Autodesk Fusion 360 part; units mm, degrees
(part 3 of 23)
  arc A1021 (27.2288, 53.8875) -> (27.2288, 53.8367) centre (27.2288, 53.8621) ccw
  arc A1022 (31.8008, 2.5146) -> (31.8008, 2.4638) centre (31.8008, 2.4892) ccw
  arc A1023 (65.6214, 47.9446) -> (65.5634, 47.994) centre (65.5924, 47.9693) ccw
  arc A1024 (33.504, 1.5804) -> (33.4532, 1.5804) centre (33.4786, 1.5804) ccw
  arc A1025 (34.1907, 2.4638) -> (34.1907, 2.5146) centre (34.1907, 2.4892) ccw
  arc A1026 (34.4504, 2.4638) -> (34.4504, 2.5146) centre (34.4504, 2.4892) ccw
  arc A1027 (32.4499, 2.4638) -> (32.4499, 2.5146) centre (32.4499, 2.4892) ccw
  arc A1028 (33.219, 1.3462) -> (33.219, 1.2954) centre (33.219, 1.3208) ccw
  arc A1029 (33.4532, 1.5804) -> (33.504, 1.5804) centre (33.4786, 1.5804) ccw
  arc A1030 (65.766, 48.2854) -> (65.6898, 48.2854) centre (65.7279, 48.2854) ccw
  arc A1031 (65.7279, 47.0281) -> (65.7279, 47.1043) centre (65.7279, 47.0662) ccw
  arc A1032 (32.8873, 2.2296) -> (32.8366, 2.2296) centre (32.862, 2.2296) ccw
  line L321 (64.8248, 47.0662) -> (65.7279, 47.0662)
  arc A1033 (33.3366, 1.7853) -> (33.3609, 1.8299) centre (33.3488, 1.8076) ccw
  line L322 (34.4504, 1.3208) -> (34.1907, 1.3208)
  arc A1034 (64.8248, 47.1043) -> (64.8248, 47.0281) centre (64.8248, 47.0662) ccw
  arc A1035 (33.9565, 2.2296) -> (33.9057, 2.2296) centre (33.9311, 2.2296) ccw
  arc A1036 (32.9789, 1.9805) -> (33.0047, 2.0242) centre (32.9918, 2.0023) ccw
  arc A1037 (33.1216, 2.4892) -> (32.862, 2.2296) centre (33.1216, 2.2296) ccw
  arc A1038 (33.4786, 1.5804) -> (33.3488, 1.8076) centre (33.2149, 1.5804) ccw
  arc A1039 (34.1907, 1.2954) -> (34.1907, 1.3462) centre (34.1907, 1.3208) ccw
  arc A1040 (32.1, 1.3208) -> (32.1508, 1.3208) centre (32.1254, 1.3208) ccw
  arc A1041 (33.219, 1.2954) -> (33.219, 1.3462) centre (33.219, 1.3208) ccw
  arc A1042 (33.1216, 2.5146) -> (33.1216, 2.4638) centre (33.1216, 2.4892) ccw
  arc A1043 (33.9057, 1.5804) -> (33.9565, 1.5804) centre (33.9311, 1.5804) ccw
  arc A1044 (33.9057, 2.2296) -> (33.9565, 2.2296) centre (33.9311, 2.2296) ccw
  arc A1045 (34.1907, 2.4892) -> (33.9311, 2.2296) centre (34.1907, 2.2296) ccw
  line L323 (34.1907, 2.4892) -> (34.4504, 2.4892)
  arc A1046 (34.871, 2.2494) -> (34.9028, 2.2097) centre (34.8869, 2.2295) ccw
  line L324 (34.8869, 2.2296) -> (35.2114, 2.4892)
  arc A1047 (35.2368, 2.4892) -> (35.186, 2.4892) centre (35.2114, 2.4892) ccw
  arc A1048 (32.8475, 1.501) -> (32.8115, 1.4652) centre (32.8295, 1.4831) ccw
  arc A1049 (32.8366, 2.2296) -> (32.8873, 2.2296) centre (32.862, 2.2296) ccw
  arc A1050 (34.8869, 1.3462) -> (34.8869, 1.2954) centre (34.8869, 1.3208) ccw
  line L325 (32.1254, 1.3208) -> (32.1254, 2.4892)
  line L326 (36.0299, 2.2296) -> (36.3544, 2.4892)
  line L327 (65.5924, 47.9693) -> (64.8248, 47.0662)
  line L328 (34.8869, 1.3208) -> (35.536, 1.3208)
  arc A1051 (36.3703, 2.4694) -> (36.3386, 2.509) centre (36.3544, 2.4892) ccw
  arc A1052 (36.014, 2.2494) -> (36.0458, 2.2097) centre (36.0299, 2.2295) ccw
  line L329 (31.8008, 2.4892) -> (32.4499, 2.4892)
  arc A1053 (33.9311, 1.5804) -> (34.1907, 1.3208) centre (34.1907, 1.5804) ccw
  arc A1054 (33.1216, 2.4638) -> (33.1216, 2.5146) centre (33.1216, 2.4892) ccw
  arc A1055 (33.3985, 2.3715) -> (33.4289, 2.4122) centre (33.4137, 2.3918) ccw
  line L330 (33.3488, 1.8076) -> (32.9918, 2.0024)
  arc A1056 (35.2273, 2.4694) -> (35.1956, 2.509) centre (35.2114, 2.4892) ccw
  line L331 (36.3544, 2.4892) -> (36.3544, 1.3208)
  arc A1057 (34.4504, 1.2954) -> (34.4504, 1.3462) centre (34.4504, 1.3208) ccw
  arc A1058 (33.219, 1.3208) -> (33.4786, 1.5804) centre (33.219, 1.5804) ccw
  arc A1059 (64.7957, 47.0909) -> (64.8538, 47.0415) centre (64.8247, 47.0662) ccw
  arc A1060 (32.1508, 2.4892) -> (32.1, 2.4892) centre (32.1254, 2.4892) ccw
  line L332 (33.9311, 1.5804) -> (33.9311, 2.2296)
  arc A1061 (53.8714, 1.9445) -> (53.8714, 1.9953) centre (53.8714, 1.9699) ccw
  arc A1062 (34.1907, 1.3462) -> (34.1907, 1.2954) centre (34.1907, 1.3208) ccw
  line L333 (54.9481, 1.3208) -> (54.6885, 1.3208)
  arc A1063 (33.0039, 2.0247) -> (32.9796, 1.9801) centre (32.9917, 2.0024) ccw
  arc A1064 (33.4137, 2.3918) -> (33.1216, 2.4892) centre (33.1216, 2.0024) ccw
  arc A1065 (34.1907, 2.5146) -> (34.1907, 2.4638) centre (34.1907, 2.4892) ccw
  arc A1066 (35.186, 1.3208) -> (35.2368, 1.3208) centre (35.2114, 1.3208) ccw
  arc A1067 (35.536, 1.2954) -> (35.536, 1.3462) centre (35.536, 1.3208) ccw
  arc A1068 (32.862, 2.2296) -> (32.9918, 2.0024) centre (33.1257, 2.2296) ccw
  arc A1069 (33.3617, 1.8295) -> (33.3359, 1.7857) centre (33.3488, 1.8076) ccw
  arc A1070 (32.8295, 1.4831) -> (33.219, 1.3208) centre (33.219, 1.8694) ccw
  arc A1071 (33.9565, 1.5804) -> (33.9057, 1.5804) centre (33.9311, 1.5804) ccw
  line L334 (35.2114, 2.4892) -> (35.2114, 1.3208)
  line L335 (59.134, 11.2155) -> (57.706, 11.7348)
  line L336 (34.2251, 29.7505) -> (34.8742, 29.1987)
  arc A1072 (33.9576, 29.1745) -> (33.9733, 29.2229) centre (33.9655, 29.1987) ccw
  line L337 (55.633, 1.3208) -> (55.633, 2.4892)
  arc A1073 (26.6305, 29.6644) -> (26.5797, 29.6644) centre (26.6051, 29.6644) ccw
  arc A1074 (50.9947, 29.8986) -> (50.9947, 29.9494) centre (50.9947, 29.924) ccw
  arc A1075 (55.6584, 2.4892) -> (55.6076, 2.4892) centre (55.633, 2.4892) ccw
  arc A1076 (58.9788, 10.1219) -> (59.0296, 10.1219) centre (59.0042, 10.1219) ccw
  arc A1077 (59.1253, 11.1916) -> (59.1427, 11.2394) centre (59.134, 11.2155) ccw
  arc A1078 (57.8499, 14.0955) -> (57.8217, 14.0533) centre (57.8358, 14.0744) ccw
  arc A1079 (59.0156, 12.8511) -> (58.9928, 12.8966) centre (59.0042, 12.8739) ccw
  arc A1080 (58.9901, 13.2743) -> (59.0183, 13.3166) centre (59.0042, 13.2954) ccw
  arc A1081 (36.679, 1.2954) -> (36.679, 1.3462) centre (36.679, 1.3208) ccw
  arc A1082 (57.8217, 13.3166) -> (57.8499, 13.2743) centre (57.8358, 13.2954) ccw
  arc A1083 (60.3758, 8.9662) -> (60.3758, 8.9154) centre (60.3758, 8.9408) ccw
  arc A1084 (60.7004, 9.5899) -> (60.3758, 9.2654) centre (60.7004, 9.2653) ccw
  arc A1085 (58.5103, 12.5493) -> (58.4595, 12.5493) centre (58.4849, 12.5493) ccw
  arc A1086 (57.8104, 12.2248) -> (57.8612, 12.2248) centre (57.8358, 12.2248) ccw
  line L338 (54.6885, 2.4892) -> (54.9481, 2.4892)
  arc A1087 (57.8104, 12.5493) -> (57.8612, 12.5493) centre (57.8358, 12.5493) ccw
  line L339 (58.4849, 12.5493) -> (58.4849, 12.2248)
  line L340 (59.0042, 12.2248) -> (57.8358, 12.2248)
  line L341 (61.5442, 8.9408) -> (60.3758, 8.9408)
  arc A1088 (60.7004, 9.5645) -> (60.7004, 9.6153) centre (60.7004, 9.5899) ccw
  arc A1089 (54.6885, 1.2954) -> (54.6885, 1.3462) centre (54.6885, 1.3208) ccw
  arc A1090 (53.4819, 1.9953) -> (53.4819, 1.9445) centre (53.4819, 1.9699) ccw
  arc A1091 (60.3504, 9.2654) -> (60.4012, 9.2654) centre (60.3758, 9.2654) ccw
  line L342 (60.7004, 9.5899) -> (61.2196, 9.5899)
  arc A1092 (60.3504, 8.9408) -> (60.4012, 8.9408) centre (60.3758, 8.9408) ccw
  arc A1093 (50.9947, 29.924) -> (50.7351, 29.6644) centre (50.9947, 29.6644) ccw
  arc A1094 (59.0042, 12.1994) -> (59.0042, 12.2502) centre (59.0042, 12.2248) ccw
  arc A1095 (54.4034, 2.2296) -> (54.4542, 2.2296) centre (54.4288, 2.2296) ccw
  arc A1096 (34.2067, 29.7329) -> (34.2435, 29.768) centre (34.2251, 29.7505) ccw
  arc A1097 (58.4849, 12.5493) -> (57.8358, 12.5493) centre (58.1604, 12.5493) ccw
  arc A1098 (26.5797, 29.6644) -> (26.6305, 29.6644) centre (26.6051, 29.6644) ccw
  arc A1099 (61.5188, 9.2654) -> (61.5696, 9.2654) centre (61.5442, 9.2654) ccw
  arc A1100 (36.3798, 2.4892) -> (36.329, 2.4892) centre (36.3544, 2.4892) ccw
  arc A1101 (60.7004, 9.6153) -> (60.7004, 9.5645) centre (60.7004, 9.5899) ccw
  arc A1102 (60.5492, 10.2421) -> (60.5269, 10.1964) centre (60.5381, 10.2192) ccw
  arc A1103 (60.4012, 9.2654) -> (60.3504, 9.2654) centre (60.3758, 9.2654) ccw
  arc A1104 (61.2196, 9.5645) -> (61.2196, 9.6153) centre (61.2196, 9.5899) ccw
  line L343 (57.8358, 12.2248) -> (57.8358, 12.5493)
  arc A1105 (57.8612, 12.5493) -> (57.8104, 12.5493) centre (57.8358, 12.5493) ccw
  line L344 (59.0042, 12.8739) -> (58.4849, 12.6142)
  arc A1106 (33.6978, 28.4044) -> (33.7138, 28.3562) centre (33.7058, 28.3803) ccw
  line L345 (61.5442, 9.2654) -> (61.5442, 8.9408)
  arc A1107 (33.9979, 29.8224) -> (33.9979, 29.8732) centre (33.9979, 29.8478) ccw
  line L346 (60.3758, 8.9408) -> (60.3758, 9.2654)
  arc A1108 (33.7312, 29.5557) -> (33.6804, 29.5557) centre (33.7058, 29.5557) ccw
  arc A1109 (61.5442, 8.9154) -> (61.5442, 8.9662) centre (61.5442, 8.9408) ccw
  arc A1110 (34.2251, 29.7505) -> (33.9979, 29.8478) centre (33.998, 29.5341) ccw
  arc A1111 (33.7058, 29.5557) -> (33.9654, 29.1987) centre (34.081, 29.5557) ccw
  line L347 (57.8358, 13.2955) -> (59.0042, 14.0744)
  arc A1112 (61.5188, 8.9408) -> (61.5696, 8.9408) centre (61.5442, 8.9408) ccw
  arc A1113 (57.7147, 11.7587) -> (57.6973, 11.7109) centre (57.706, 11.7348) ccw
  arc A1114 (58.4595, 12.5493) -> (58.5103, 12.5493) centre (58.4849, 12.5493) ccw
  arc A1115 (58.4736, 12.6369) -> (58.4963, 12.5915) centre (58.4849, 12.6142) ccw
  arc A1116 (61.5442, 9.2654) -> (61.2196, 9.5899) centre (61.2196, 9.2653) ccw
  arc A1117 (59.0296, 10.771) -> (58.9788, 10.771) centre (59.0042, 10.771) ccw
  arc A1118 (58.4595, 12.2248) -> (58.5103, 12.2248) centre (58.4849, 12.2248) ccw
  line L348 (59.0042, 13.2955) -> (57.8358, 14.0744)
  arc A1119 (57.8358, 12.2502) -> (57.8358, 12.1994) centre (57.8358, 12.2248) ccw
  arc A1120 (59.0183, 14.0533) -> (58.9901, 14.0955) centre (59.0042, 14.0744) ccw
  arc A1121 (61.2196, 9.6153) -> (61.2196, 9.5645) centre (61.2196, 9.5899) ccw
  arc A1122 (60.3504, 10.4464) -> (60.4012, 10.4465) centre (60.3758, 10.4465) ccw
  arc A1123 (61.3737, 10.2433) -> (61.3902, 10.1952) centre (61.382, 10.2192) ccw
  arc A1124 (60.3504, 12.1031) -> (60.4012, 12.1031) centre (60.3758, 12.1031) ccw
  arc A1125 (61.5301, 13.0838) -> (61.5583, 13.1261) centre (61.5442, 13.105) ccw
  arc A1126 (43.4975, 9.6224) -> (43.4467, 9.6224) centre (43.4721, 9.6224) ccw
  arc A1127 (61.5696, 10.4464) -> (61.5188, 10.4465) centre (61.5442, 10.4465) ccw
  arc A1128 (60.6513, 10.7259) -> (60.6196, 10.6863) centre (60.6354, 10.7061) ccw
  arc A1129 (60.2547, 11.7587) -> (60.2373, 11.7109) centre (60.246, 11.7348) ccw
  arc A1130 (60.4012, 12.7522) -> (60.3504, 12.7522) centre (60.3758, 12.7522) ccw
  line L349 (60.3758, 13.105) -> (61.5442, 13.8839)
  arc A1131 (42.6212, 10.4733) -> (42.5704, 10.4733) centre (42.5958, 10.4733) ccw
  line L350 (61.5442, 13.105) -> (60.3758, 13.8839)
  arc A1132 (61.3931, 10.1964) -> (61.3708, 10.2421) centre (61.382, 10.2192) ccw
  arc A1133 (60.96, 10.7456) -> (60.96, 10.7964) centre (60.96, 10.771) ccw
  arc A1134 (60.5381, 10.2193) -> (60.96, 10.1219) centre (60.9601, 11.0846) ccw
  arc A1135 (60.96, 10.0965) -> (60.96, 10.1473) centre (60.96, 10.1219) ccw
  arc A1136 (61.6653, 11.1916) -> (61.6827, 11.2394) centre (61.674, 11.2155) ccw
  arc A1137 (61.3708, 10.6508) -> (61.3931, 10.6965) centre (61.382, 10.6737) ccw
  line L351 (61.5442, 12.4276) -> (60.3758, 12.4276)
  arc A1138 (61.5583, 13.8628) -> (61.5301, 13.905) centre (61.5442, 13.8839) ccw
  arc A1139 (60.5381, 10.6736) -> (60.3758, 10.4465) centre (60.6159, 10.4465) ccw
  arc A1140 (60.3617, 13.1261) -> (60.3899, 13.0838) centre (60.3758, 13.1049) ccw
  line L352 (43.4721, 9.6224) -> (43.4721, 9.0382)
  arc A1141 (60.3758, 10.4465) -> (60.5381, 10.2193) centre (60.616, 10.4465) ccw
  arc A1142 (43.7722, 9.6956) -> (43.7562, 9.7438) centre (43.7642, 9.7197) ccw
  arc A1143 (42.5878, 9.3544) -> (42.6038, 9.3062) centre (42.5958, 9.3303) ccw
  arc A1144 (60.5463, 10.6496) -> (60.5298, 10.6977) centre (60.5381, 10.6737) ccw
  arc A1145 (61.5442, 10.4465) -> (61.3819, 10.6736) centre (61.3041, 10.4465) ccw
  arc A1146 (42.7692, 10.2689) -> (42.7469, 10.2232) centre (42.758, 10.246) ccw
  arc A1147 (42.7581, 10.7005) -> (42.5958, 10.4733) centre (42.836, 10.4733) ccw
  arc A1148 (43.18, 10.7978) -> (42.7581, 10.7005) centre (43.1798, 9.8351) ccw
  arc A1149 (60.96, 10.1219) -> (61.3819, 10.2193) centre (60.9599, 11.0846) ccw
  arc A1150 (61.5696, 9.2654) -> (61.5188, 9.2654) centre (61.5442, 9.2654) ccw
  arc A1151 (60.96, 10.1473) -> (60.96, 10.0965) centre (60.96, 10.1219) ccw
  arc A1152 (60.3899, 13.905) -> (60.3617, 13.8628) centre (60.3758, 13.8839) ccw
  arc A1153 (60.96, 10.7964) -> (60.96, 10.7456) centre (60.96, 10.771) ccw
  line L353 (42.5958, 9.3303) -> (43.7642, 9.7197)
  arc A1154 (60.3758, 12.453) -> (60.3758, 12.4022) centre (60.3758, 12.4276) ccw
  arc A1155 (42.5958, 10.4733) -> (42.7581, 10.2461) centre (42.836, 10.4733) ccw
  arc A1156 (61.3819, 10.6736) -> (60.96, 10.771) centre (60.9599, 9.8083) ccw
  arc A1157 (42.6038, 9.3544) -> (42.5878, 9.3062) centre (42.5958, 9.3303) ccw
  arc A1158 (61.3902, 10.6977) -> (61.3737, 10.6496) centre (61.382, 10.6737) ccw
  arc A1159 (42.5704, 10.4733) -> (42.6212, 10.4733) centre (42.5958, 10.4733) ccw
  arc A1160 (42.7469, 10.7233) -> (42.7692, 10.6776) centre (42.758, 10.7005) ccw
  arc A1161 (61.5188, 10.4464) -> (61.5696, 10.4465) centre (61.5442, 10.4465) ccw
  arc A1162 (42.7581, 10.2461) -> (43.18, 10.1487) centre (43.1801, 11.1114) ccw
  arc A1163 (60.5269, 10.6965) -> (60.5492, 10.6508) centre (60.5381, 10.6737) ccw
  arc A1164 (61.2687, 10.167) -> (61.3004, 10.2066) centre (61.2846, 10.1868) ccw
  line L354 (61.2846, 10.1868) -> (60.6354, 10.7061)
  arc A1165 (60.96, 10.771) -> (60.5381, 10.6736) centre (60.9601, 9.8083) ccw
  arc A1166 (61.5442, 12.4022) -> (61.5442, 12.453) centre (61.5442, 12.4276) ccw
  line L355 (60.3758, 12.1031) -> (60.3758, 12.7522)
  arc A1167 (60.4012, 10.4464) -> (60.3504, 10.4465) centre (60.3758, 10.4465) ccw
  line L356 (43.7642, 8.9408) -> (42.5958, 9.3303)
  arc A1168 (60.5298, 10.1952) -> (60.5463, 10.2433) centre (60.5381, 10.2193) ccw
  arc A1169 (43.7562, 8.9167) -> (43.7722, 8.9649) centre (43.7642, 8.9408) ccw
  arc A1170 (43.4467, 9.0382) -> (43.4975, 9.0382) centre (43.4721, 9.0382) ccw
  arc A1171 (42.7498, 10.222) -> (42.7663, 10.2701) centre (42.758, 10.2461) ccw
  arc A1172 (43.18, 10.1233) -> (43.18, 10.1741) centre (43.18, 10.1487) ccw
  line L357 (61.674, 11.2155) -> (60.246, 11.7348)
  arc A1173 (42.7663, 10.6764) -> (42.7498, 10.7245) centre (42.758, 10.7005) ccw
  arc A1174 (43.18, 10.1741) -> (43.18, 10.1233) centre (43.18, 10.1487) ccw
  arc A1175 (61.3819, 10.2193) -> (61.5442, 10.4465) centre (61.304, 10.4465) ccw
  arc A1176 (43.6131, 10.2232) -> (43.5908, 10.2689) centre (43.602, 10.2461) ccw
  arc A1177 (43.18, 10.1487) -> (43.6019, 10.2461) centre (43.1799, 11.1114) ccw
  arc A1178 (43.6019, 10.2461) -> (43.7642, 10.4733) centre (43.524, 10.4733) ccw
  arc A1179 (43.7388, 10.4733) -> (43.7896, 10.4733) centre (43.7642, 10.4733) ccw
  line L358 (55.9774, 12.6873) -> (55.7826, 12.3303)
  arc A1180 (56.4896, 13.7889) -> (56.4388, 13.7889) centre (56.4642, 13.7889) ccw
  arc A1181 (45.1358, 10.4987) -> (45.1358, 10.4479) centre (45.1358, 10.4733) ccw
  arc A1182 (55.4135, 12.737) -> (55.3728, 12.7674) centre (55.3932, 12.7522) ccw
  arc A1183 (45.1278, 9.3544) -> (45.1438, 9.3062) centre (45.1358, 9.3303) ccw
  arc A1184 (42.8713, 10.7527) -> (42.8396, 10.7131) centre (42.8554, 10.7329) ccw
  arc A1185 (45.1556, 10.4891) -> (45.116, 10.4574) centre (45.1358, 10.4732) ccw
  line L359 (45.3954, 10.1487) -> (45.1358, 10.4733)
  arc A1186 (43.18, 10.8232) -> (43.18, 10.7724) centre (43.18, 10.7978) ccw
  arc A1187 (46.2962, 8.9167) -> (46.3122, 8.9649) centre (46.3042, 8.9408) ccw
  line L360 (45.1358, 9.3303) -> (46.3042, 9.7197)
  line L361 (46.3042, 10.1487) -> (46.3042, 10.7978)
  arc A1188 (48.8522, 9.6956) -> (48.8362, 9.7438) centre (48.8442, 9.7197) ccw
  arc A1189 (56.4388, 13.5292) -> (56.4896, 13.5292) centre (56.4642, 13.5292) ccw
  arc A1190 (48.8362, 8.9167) -> (48.8522, 8.9649) centre (48.8442, 8.9408) ccw
  arc A1191 (47.6838, 9.3544) -> (47.6678, 9.3062) centre (47.6758, 9.3303) ccw
  arc A1192 (48.5775, 9.6224) -> (48.5267, 9.6224) centre (48.5521, 9.6224) ccw
  arc A1193 (56.2046, 13.2696) -> (56.4642, 13.5292) centre (56.2046, 13.5292) ccw
  arc A1194 (56.2046, 13.295) -> (56.2046, 13.2442) centre (56.2046, 13.2696) ccw
  arc A1195 (46.3122, 9.6956) -> (46.2962, 9.7438) centre (46.3042, 9.7197) ccw
  arc A1196 (45.3756, 10.1328) -> (45.4153, 10.1646) centre (45.3955, 10.1487) ccw
  line L362 (43.5046, 10.2136) -> (42.8554, 10.7329)
  arc A1197 (43.5937, 10.2701) -> (43.6102, 10.222) centre (43.602, 10.246) ccw
  arc A1198 (43.7642, 10.4733) -> (43.6019, 10.7005) centre (43.524, 10.4733) ccw
  line L363 (46.3042, 8.9408) -> (45.1358, 9.3303)
  arc A1199 (43.4887, 10.1938) -> (43.5204, 10.2335) centre (43.5045, 10.2137) ccw
  arc A1200 (54.6885, 2.4892) -> (54.4288, 2.2296) centre (54.6885, 2.2295) ccw
  arc A1201 (46.2788, 10.1487) -> (46.3296, 10.1487) centre (46.3042, 10.1487) ccw
  arc A1202 (56.2046, 12.8171) -> (55.9774, 12.6873) centre (56.2046, 12.5534) ccw
  line L364 (56.4642, 13.7889) -> (56.4642, 13.5292)
  arc A1203 (46.3296, 10.7978) -> (46.2788, 10.7978) centre (46.3042, 10.7978) ccw
  line L365 (47.6758, 9.3303) -> (48.8442, 9.7197)
  arc A1204 (45.9867, 9.0382) -> (46.0375, 9.0382) centre (46.0121, 9.0382) ccw
  line L366 (48.8442, 8.9408) -> (47.6758, 9.3303)
  arc A1205 (43.7896, 10.4733) -> (43.7388, 10.4733) centre (43.7642, 10.4733) ccw
  line L367 (27.2542, 30.7425) -> (26.0858, 31.1319)
  arc A1206 (43.5908, 10.6776) -> (43.6131, 10.7233) centre (43.602, 10.7005) ccw
  arc A1207 (43.6019, 10.7005) -> (43.18, 10.7978) centre (43.1802, 9.8351) ccw
  arc A1208 (43.6102, 10.7245) -> (43.5937, 10.6764) centre (43.602, 10.7005) ccw
  line L368 (46.0121, 9.6224) -> (46.0121, 9.0382)
  arc A1209 (45.1438, 9.3544) -> (45.1278, 9.3062) centre (45.1358, 9.3303) ccw
  arc A1210 (46.3042, 10.4479) -> (46.3042, 10.4987) centre (46.3042, 10.4733) ccw
  arc A1211 (47.6678, 9.3544) -> (47.6838, 9.3062) centre (47.6758, 9.3303) ccw
  arc A1212 (47.9679, 10.7978) -> (47.6758, 10.5057) centre (47.9679, 10.5057) ccw
  arc A1213 (26.8647, 29.9494) -> (26.8647, 29.8986) centre (26.8647, 29.924) ccw
  arc A1214 (55.2704, 12.4601) -> (55.3212, 12.4601) centre (55.2958, 12.4601) ccw
  arc A1215 (55.8045, 12.3174) -> (55.7608, 12.3432) centre (55.7827, 12.3303) ccw
  arc A1216 (46.0375, 9.6224) -> (45.9867, 9.6224) centre (46.0121, 9.6224) ccw
  line L369 (48.5521, 9.6224) -> (48.5521, 9.0382)
  arc A1217 (26.6051, 29.2495) -> (26.6051, 29.3003) centre (26.6051, 29.2749) ccw
  arc A1218 (29.7688, 28.2504) -> (29.8196, 28.2504) centre (29.7942, 28.2504) ccw
  arc A1219 (55.9997, 12.6751) -> (55.9551, 12.6995) centre (55.9774, 12.6873) ccw
  arc A1220 (56.2046, 12.7917) -> (56.2046, 12.8425) centre (56.2046, 12.8171) ccw
  arc A1221 (48.5267, 9.0382) -> (48.5775, 9.0382) centre (48.5521, 9.0382) ccw
  arc A1222 (43.18, 10.7724) -> (43.18, 10.8232) centre (43.18, 10.7978) ccw
  line L370 (45.1358, 10.4733) -> (46.3042, 10.4733)
  arc A1223 (55.9555, 12.7002) -> (55.9993, 12.6744) centre (55.9774, 12.6873) ccw
  arc A1224 (55.5554, 12.2005) -> (55.7826, 12.3303) centre (55.5554, 12.4642) ccw
  arc A1225 (55.5554, 12.2259) -> (55.5554, 12.1751) centre (55.5554, 12.2005) ccw
  arc A1226 (55.7603, 12.3424) -> (55.8049, 12.3181) centre (55.7826, 12.3302) ccw
  arc A1227 (56.4896, 13.5292) -> (56.4388, 13.5292) centre (56.4642, 13.5292) ccw
  arc A1228 (35.7547, 10.8486) -> (35.7547, 10.8994) centre (35.7547, 10.874) ccw
  arc A1229 (35.6644, 8.9408) -> (35.7152, 8.9408) centre (35.6898, 8.9408) ccw
  line L371 (33.5393, 9.3303) -> (32.7604, 9.3303)
  arc A1230 (33.1244, 8.9408) -> (33.1752, 8.9408) centre (33.1498, 8.9408) ccw
  line L372 (33.6042, 11.6925) -> (32.4358, 12.0819)
  arc A1231 (32.9297, 10.2249) -> (32.9805, 10.2249) centre (32.9551, 10.2249) ccw
  line L373 (33.6042, 10.2249) -> (33.6042, 10.6144)
  arc A1232 (55.3212, 13.5292) -> (55.2704, 13.5292) centre (55.2958, 13.5292) ccw
  arc A1233 (35.3004, 9.3557) -> (35.3004, 9.3049) centre (35.3004, 9.3303) ccw
  arc A1234 (33.1752, 9.7197) -> (33.1244, 9.7197) centre (33.1498, 9.7197) ccw
  line L374 (32.9551, 10.6144) -> (32.9551, 10.2249)
  arc A1235 (55.2704, 13.5292) -> (55.3212, 13.5292) centre (55.2958, 13.5292) ccw
  arc A1236 (56.4642, 14.2404) -> (56.4642, 14.2912) centre (56.4642, 14.2658) ccw
  arc A1237 (56.4896, 14.7851) -> (56.4388, 14.7851) centre (56.4642, 14.7851) ccw
  arc A1238 (56.2046, 13.2442) -> (56.2046, 13.295) centre (56.2046, 13.2696) ccw
  line L375 (56.2046, 13.2696) -> (55.5554, 13.2696)
  arc A1239 (56.4388, 14.2658) -> (56.4896, 14.2658) centre (56.4642, 14.2658) ccw
  arc A1240 (32.9551, 10.1995) -> (32.9551, 10.2503) centre (32.9551, 10.2249) ccw
  line L376 (56.4642, 14.2658) -> (56.4642, 14.7851)
  arc A1241 (32.4438, 12.106) -> (32.4278, 12.0578) centre (32.4358, 12.0819) ccw
  line L377 (36.0793, 9.3303) -> (35.3004, 9.3303)
  line L378 (36.1442, 10.2249) -> (36.1442, 10.6144)
  arc A1242 (36.1696, 10.6144) -> (36.1188, 10.6144) centre (36.1442, 10.6144) ccw
  line L379 (35.8846, 10.874) -> (35.7547, 10.874)
  line L380 (33.1498, 8.9408) -> (33.1498, 9.7197)
  arc A1243 (33.5788, 10.2249) -> (33.6296, 10.2249) centre (33.6042, 10.2249) ccw
  arc A1244 (33.5788, 10.6144) -> (33.6296, 10.6144) centre (33.6042, 10.6144) ccw
  arc A1245 (33.2147, 10.8994) -> (33.2147, 10.8486) centre (33.2147, 10.874) ccw
  arc A1246 (32.4278, 11.3271) -> (32.4438, 11.2789) centre (32.4358, 11.303) ccw
  line L381 (32.4358, 10.2249) -> (32.4358, 10.874)
  line L382 (35.6898, 8.9408) -> (35.6898, 9.7197)
  line L383 (32.4358, 11.303) -> (33.6042, 11.6925)
  line L384 (32.9551, 10.2249) -> (32.4358, 10.2249)
  arc A1247 (35.7547, 10.8994) -> (35.7547, 10.8486) centre (35.7547, 10.874) ccw
  arc A1248 (36.0793, 9.3049) -> (36.0793, 9.3557) centre (36.0793, 9.3303) ccw
  arc A1249 (35.8846, 10.8486) -> (35.8846, 10.8994) centre (35.8846, 10.874) ccw
  line L385 (33.3446, 10.874) -> (33.2147, 10.874)
  arc A1250 (32.9805, 10.6144) -> (32.9297, 10.6144) centre (32.9551, 10.6144) ccw
  arc A1251 (32.4358, 10.2503) -> (32.4358, 10.1995) centre (32.4358, 10.2249) ccw
  line L386 (55.2958, 13.5292) -> (55.2958, 13.7889)
  arc A1252 (33.5393, 9.3049) -> (33.5393, 9.3557) centre (33.5393, 9.3303) ccw
  arc A1253 (55.5554, 13.295) -> (55.5554, 13.2442) centre (55.5554, 13.2696) ccw
  arc A1254 (33.2147, 10.8486) -> (33.2147, 10.8994) centre (33.2147, 10.874) ccw
  arc A1255 (33.2147, 10.874) -> (32.9551, 10.6144) centre (33.2147, 10.6144) ccw
  arc A1256 (33.3446, 10.8994) -> (33.3446, 10.8486) centre (33.3446, 10.874) ccw
  arc A1257 (35.7152, 9.7197) -> (35.6644, 9.7197) centre (35.6898, 9.7197) ccw
  line L387 (55.2958, 14.2658) -> (56.4642, 14.2658)
  arc A1258 (32.4612, 10.874) -> (32.4104, 10.874) centre (32.4358, 10.874) ccw
  arc A1259 (55.2958, 14.2912) -> (55.2958, 14.2404) centre (55.2958, 14.2658) ccw
  arc A1260 (33.6122, 11.6684) -> (33.5962, 11.7166) centre (33.6042, 11.6925) ccw
  arc A1261 (32.4104, 10.2249) -> (32.4612, 10.2249) centre (32.4358, 10.2249) ccw
  arc A1262 (33.5962, 11.6684) -> (33.6122, 11.7166) centre (33.6042, 11.6925) ccw
  arc A1263 (55.3212, 13.7889) -> (55.2704, 13.7889) centre (55.2958, 13.7889) ccw
  arc A1264 (36.1188, 10.6144) -> (36.1696, 10.6144) centre (36.1442, 10.6144) ccw
  arc A1265 (55.2958, 13.5292) -> (55.5554, 13.2696) centre (55.5554, 13.5292) ccw
  arc A1266 (33.6296, 10.6144) -> (33.5788, 10.6144) centre (33.6042, 10.6144) ccw
  arc A1267 (33.3446, 10.8486) -> (33.3446, 10.8994) centre (33.3446, 10.874) ccw
  arc A1268 (32.9297, 10.6144) -> (32.9805, 10.6144) centre (32.9551, 10.6144) ccw
  arc A1269 (36.1442, 10.6144) -> (35.8846, 10.874) centre (35.8846, 10.6144) ccw
  arc A1270 (36.1188, 10.2249) -> (36.1696, 10.2249) centre (36.1442, 10.2249) ccw
  arc A1271 (55.5554, 13.2442) -> (55.5554, 13.295) centre (55.5554, 13.2696) ccw
  arc A1272 (33.6042, 10.6144) -> (33.3446, 10.874) centre (33.3446, 10.6144) ccw
  arc A1273 (32.7604, 9.3557) -> (32.7604, 9.3049) centre (32.7604, 9.3303) ccw
  arc A1274 (35.8846, 10.8994) -> (35.8846, 10.8486) centre (35.8846, 10.874) ccw
  line L388 (35.4951, 10.6144) -> (35.4951, 10.2249)
  line L389 (34.9758, 10.2249) -> (34.9758, 10.874)
  arc A1275 (37.5412, 9.2004) -> (37.4904, 9.2004) centre (37.5158, 9.2004) ccw
  arc A1276 (37.5412, 9.5899) -> (37.4904, 9.5899) centre (37.5158, 9.5899) ccw
  arc A1277 (37.8404, 12.0283) -> (37.5158, 11.7037) centre (37.8404, 11.7037) ccw
  arc A1278 (35.4697, 10.2249) -> (35.5205, 10.2249) centre (35.4951, 10.2249) ccw
  arc A1279 (35.5205, 10.6144) -> (35.4697, 10.6144) centre (35.4951, 10.6144) ccw
  line L390 (38.0351, 9.5899) -> (38.6842, 9.5899)
  arc A1280 (38.0351, 9.6153) -> (38.0351, 9.5645) centre (38.0351, 9.5899) ccw
  arc A1281 (38.6842, 10.1346) -> (38.6842, 10.1854) centre (38.6842, 10.16) ccw
  line L391 (38.6842, 9.5899) -> (38.6842, 9.2004)
  arc A1282 (37.5158, 11.4046) -> (37.5158, 11.3538) centre (37.5158, 11.3792) ccw
  arc A1283 (38.6842, 11.7037) -> (38.3596, 12.0283) centre (38.3596, 11.7037) ccw
  arc A1284 (38.3596, 12.0029) -> (38.3596, 12.0537) centre (38.3596, 12.0283) ccw
  line L392 (37.5158, 9.2004) -> (37.5158, 9.5899)
  line L393 (37.5158, 10.16) -> (38.6842, 10.8091)
  arc A1285 (38.0097, 9.3952) -> (38.0605, 9.3952) centre (38.0351, 9.3952) ccw
  arc A1286 (34.9504, 10.2249) -> (35.0012, 10.2249) centre (34.9758, 10.2249) ccw
  arc A1287 (38.0605, 9.5899) -> (38.0097, 9.5899) centre (38.0351, 9.5899) ccw
  arc A1288 (37.5035, 10.1822) -> (37.5281, 10.1378) centre (37.5158, 10.16) ccw
  arc A1289 (35.7547, 10.874) -> (35.4951, 10.6144) centre (35.7547, 10.6144) ccw
  arc A1290 (36.1522, 11.6684) -> (36.1362, 11.7166) centre (36.1442, 11.6925) ccw
  arc A1291 (34.9838, 12.106) -> (34.9678, 12.0578) centre (34.9758, 12.0819) ccw
  arc A1292 (37.5158, 10.8345) -> (37.5158, 10.7837) centre (37.5158, 10.8091) ccw
  arc A1293 (38.4246, 8.9408) -> (38.6842, 9.2004) centre (38.4246, 9.2004) ccw
  arc A1294 (37.4904, 9.2004) -> (37.5412, 9.2004) centre (37.5158, 9.2004) ccw
  arc A1295 (38.6842, 10.7837) -> (38.6842, 10.8345) centre (38.6842, 10.8091) ccw
  arc A1296 (38.6842, 9.5645) -> (38.6842, 9.6153) centre (38.6842, 9.5899) ccw
  arc A1297 (37.5158, 10.1854) -> (37.5158, 10.1346) centre (37.5158, 10.16) ccw
  arc A1298 (38.6965, 10.7869) -> (38.6719, 10.8313) centre (38.6842, 10.8091) ccw
  line L394 (34.9758, 11.303) -> (36.1442, 11.6925)
  arc A1299 (34.9678, 11.3271) -> (34.9838, 11.2789) centre (34.9758, 11.303) ccw
  arc A1300 (37.7754, 8.9154) -> (37.7754, 8.9662) centre (37.7754, 8.9408) ccw
  arc A1301 (35.4697, 10.6144) -> (35.5205, 10.6144) centre (35.4951, 10.6144) ccw
  arc A1302 (38.7096, 9.5899) -> (38.6588, 9.5899) centre (38.6842, 9.5899) ccw
  arc A1303 (38.4246, 8.9154) -> (38.4246, 8.9662) centre (38.4246, 8.9408) ccw
  arc A1304 (37.7754, 8.9662) -> (37.7754, 8.9154) centre (37.7754, 8.9408) ccw
  line L395 (37.5158, 11.3792) -> (37.5158, 11.7037)
  line L396 (38.6842, 10.8091) -> (37.5158, 10.8091)
  arc A1305 (35.4951, 10.1995) -> (35.4951, 10.2503) centre (35.4951, 10.2249) ccw
  line L397 (38.6842, 10.16) -> (37.5158, 10.16)
  line L398 (38.0351, 9.3952) -> (38.0351, 9.5899)
  arc A1306 (35.0012, 10.874) -> (34.9504, 10.874) centre (34.9758, 10.874) ccw
  arc A1307 (37.4904, 11.3792) -> (37.5412, 11.3792) centre (37.5158, 11.3792) ccw
  arc A1308 (37.5158, 9.2004) -> (37.7754, 8.9408) centre (37.7754, 9.2004) ccw
  arc A1309 (37.8404, 12.0029) -> (37.8404, 12.0537) centre (37.8404, 12.0283) ccw
  arc A1310 (37.5412, 11.7037) -> (37.4904, 11.7037) centre (37.5158, 11.7037) ccw
  arc A1311 (34.9758, 10.2503) -> (34.9758, 10.1995) centre (34.9758, 10.2249) ccw
  arc A1312 (38.7096, 9.2004) -> (38.6588, 9.2004) centre (38.6842, 9.2004) ccw
  arc A1313 (38.6842, 11.3538) -> (38.6842, 11.4046) centre (38.6842, 11.3792) ccw
  arc A1314 (37.4904, 11.7037) -> (37.5412, 11.7037) centre (37.5158, 11.7037) ccw
  line L399 (37.8404, 12.0283) -> (38.3596, 12.0283)
  arc A1315 (38.6588, 11.7037) -> (38.7096, 11.7037) centre (38.6842, 11.7037) ccw
  arc A1316 (38.6588, 11.3792) -> (38.7096, 11.3792) centre (38.6842, 11.3792) ccw
  line L400 (29.1451, 28.6399) -> (29.7942, 28.6399)
  line L401 (36.1442, 11.6925) -> (34.9758, 12.0819)
  arc A1317 (38.3596, 12.0537) -> (38.3596, 12.0029) centre (38.3596, 12.0283) ccw
  line L402 (38.6842, 11.3792) -> (37.5158, 11.3792)
  arc A1318 (37.8404, 12.0537) -> (37.8404, 12.0029) centre (37.8404, 12.0283) ccw
  arc A1319 (36.1362, 11.6684) -> (36.1522, 11.7166) centre (36.1442, 11.6925) ccw
  arc A1320 (38.6588, 9.2004) -> (38.7096, 9.2004) centre (38.6842, 9.2004) ccw
  line L403 (35.4951, 10.2249) -> (34.9758, 10.2249)
  arc A1321 (38.4246, 8.9662) -> (38.4246, 8.9154) centre (38.4246, 8.9408) ccw
  line L404 (38.4246, 8.9408) -> (37.7754, 8.9408)
  arc A1322 (51.1175, 9.6224) -> (51.0667, 9.6224) centre (51.0921, 9.6224) ccw
  arc A1323 (48.2115, 10.7198) -> (48.1786, 10.6811) centre (48.1951, 10.7005) ccw
  arc A1324 (50.1904, 10.5382) -> (50.2412, 10.5382) centre (50.2158, 10.5382) ccw
  arc A1325 (48.1951, 10.7005) -> (47.9679, 10.7978) centre (47.968, 10.4841) ccw
  arc A1326 (50.7605, 10.5382) -> (50.7097, 10.5382) centre (50.7351, 10.5382) ccw
  arc A1327 (50.7097, 10.2785) -> (50.7605, 10.2785) centre (50.7351, 10.2785) ccw
  line L405 (53.9242, 8.9408) -> (52.7558, 9.3303)
  arc A1328 (47.9679, 10.8232) -> (47.9679, 10.7724) centre (47.9679, 10.7978) ccw
  arc A1329 (48.1767, 10.6829) -> (48.2135, 10.718) centre (48.1951, 10.7005) ccw
  arc A1330 (48.8277, 10.1294) -> (48.8607, 10.1681) centre (48.8442, 10.1488) ccw
  line L406 (51.3842, 8.9408) -> (50.2158, 9.3303)
  line L407 (48.8442, 10.1487) -> (48.8442, 10.7978)
  arc A1331 (51.4096, 10.4733) -> (51.3588, 10.4733) centre (51.3842, 10.4733) ccw
  arc A1332 (53.9322, 9.6956) -> (53.9162, 9.7438) centre (53.9242, 9.7197) ccw
  arc A1333 (53.6575, 9.6224) -> (53.6067, 9.6224) centre (53.6321, 9.6224) ccw
  line L408 (53.6646, 10.1487) -> (53.6646, 10.7978)
  line L409 (52.7558, 10.4084) -> (53.6646, 10.1487)
  arc A1334 (51.3588, 10.1487) -> (51.4096, 10.1487) centre (51.3842, 10.1487) ccw
  line L410 (50.2158, 10.1487) -> (50.2158, 10.5382)
  arc A1335 (53.6576, 10.1243) -> (53.6715, 10.1731) centre (53.6646, 10.1487) ccw
  arc A1336 (48.8188, 10.1487) -> (48.8696, 10.1487) centre (48.8442, 10.1487) ccw
  line L411 (50.7351, 10.5382) -> (50.7351, 10.2785)
  arc A1337 (53.9162, 8.9167) -> (53.9322, 8.9649) centre (53.9242, 8.9408) ccw
  arc A1338 (50.7097, 10.5382) -> (50.7605, 10.5382) centre (50.7351, 10.5382) ccw
  line L412 (52.7558, 9.3303) -> (53.9242, 9.7197)
  arc A1339 (51.3842, 10.4733) -> (50.7351, 10.4733) centre (51.0597, 10.4733) ccw
  line L413 (48.1951, 10.7005) -> (48.8442, 10.1487)
  arc A1340 (48.8696, 10.7978) -> (48.8188, 10.7978) centre (48.8442, 10.7978) ccw
  arc A1341 (50.2078, 9.3544) -> (50.2238, 9.3062) centre (50.2158, 9.3303) ccw
  arc A1342 (50.7351, 10.5382) -> (50.2158, 10.5382) centre (50.4755, 10.5382) ccw
  line L414 (38.6842, 11.7037) -> (38.6842, 11.3792)
  arc A1343 (51.3762, 8.9167) -> (51.3922, 8.9649) centre (51.3842, 8.9408) ccw
  arc A1344 (51.3588, 10.4733) -> (51.4096, 10.4733) centre (51.3842, 10.4733) ccw
  arc A1345 (52.7638, 9.3544) -> (52.7478, 9.3062) centre (52.7558, 9.3303) ccw
  arc A1346 (50.1904, 10.1487) -> (50.2412, 10.1487) centre (50.2158, 10.1487) ccw
  arc A1347 (52.7478, 9.3544) -> (52.7638, 9.3062) centre (52.7558, 9.3303) ccw
  arc A1348 (51.3922, 9.6956) -> (51.3762, 9.7438) centre (51.3842, 9.7197) ccw
  line L415 (53.6321, 9.6224) -> (53.6321, 9.0382)
  arc A1349 (53.6067, 9.0382) -> (53.6575, 9.0382) centre (53.6321, 9.0382) ccw
  arc A1350 (50.7097, 10.4733) -> (50.7605, 10.4733) centre (50.7351, 10.4733) ccw
  arc A1351 (29.1451, 28.6653) -> (29.1451, 28.6145) centre (29.1451, 28.6399) ccw
  arc A1352 (47.7012, 10.5057) -> (47.6504, 10.5057) centre (47.6758, 10.5057) ccw
  arc A1353 (47.9276, 10.1245) -> (47.9433, 10.1729) centre (47.9355, 10.1487) ccw
  line L416 (51.0921, 9.6224) -> (51.0921, 9.0382)
  arc A1354 (51.0667, 9.0382) -> (51.1175, 9.0382) centre (51.0921, 9.0382) ccw
  arc A1355 (50.2238, 9.3544) -> (50.2078, 9.3062) centre (50.2158, 9.3303) ccw
  arc A1356 (47.6758, 10.5057) -> (47.9354, 10.1487) centre (48.051, 10.5057) ccw
  arc A1357 (29.5346, 27.9908) -> (29.7942, 28.2504) centre (29.5346, 28.2504) ccw
  line L417 (50.2158, 9.3303) -> (51.3842, 9.7197)
  arc A1358 (47.6504, 10.5057) -> (47.7012, 10.5057) centre (47.6758, 10.5057) ccw
  line L418 (51.3842, 10.1487) -> (51.3842, 10.4733)
  arc A1359 (50.2412, 10.5382) -> (50.1904, 10.5382) centre (50.2158, 10.5382) ccw
  arc A1360 (27.3304, 20.6657) -> (27.3812, 20.6657) centre (27.3558, 20.6657) ccw
  arc A1361 (41.2242, 20.2946) -> (41.2242, 20.3454) centre (41.2242, 20.32) ccw
  line L419 (40.5751, 19.7499) -> (41.2242, 19.7499)
  line L420 (25.9842, 19.1008) -> (24.8158, 19.4903)
  arc A1362 (23.0547, 21.034) -> (22.7951, 20.7744) centre (23.0547, 20.7744) ccw
  arc A1363 (27.6479, 20.9324) -> (27.6479, 20.9832) centre (27.6479, 20.9578) ccw
  arc A1364 (27.8915, 20.8798) -> (27.8586, 20.8411) centre (27.8751, 20.8605) ccw
  arc A1365 (40.3804, 22.2137) -> (40.3804, 22.1629) centre (40.3804, 22.1883) ccw
  line L421 (25.0754, 20.3087) -> (24.8158, 20.6333)
  arc A1366 (41.1988, 21.5392) -> (41.2496, 21.5392) centre (41.2242, 21.5392) ccw
  arc A1367 (41.2242, 21.5138) -> (41.2242, 21.5646) centre (41.2242, 21.5392) ccw
  line L422 (31.0642, 19.1008) -> (29.8958, 19.4903)
  arc A1368 (41.2242, 21.8637) -> (40.8996, 22.1883) centre (40.8996, 21.8637) ccw
  arc A1369 (25.9588, 20.3087) -> (26.0096, 20.3087) centre (25.9842, 20.3087) ccw
  arc A1370 (40.0558, 21.5646) -> (40.0558, 21.5138) centre (40.0558, 21.5392) ccw
  arc A1371 (40.0304, 21.8637) -> (40.0812, 21.8637) centre (40.0558, 21.8637) ccw
  line L423 (28.5242, 20.3087) -> (28.5242, 20.9578)
  arc A1372 (24.8078, 19.5144) -> (24.8238, 19.4662) centre (24.8158, 19.4903) ccw
  line L424 (22.7951, 20.7744) -> (22.7951, 20.3849)
  arc A1373 (25.9842, 20.6079) -> (25.9842, 20.6587) centre (25.9842, 20.6333) ccw
  arc A1374 (27.3812, 20.6657) -> (27.3304, 20.6657) centre (27.3558, 20.6657) ccw
  arc A1375 (29.9038, 19.5144) -> (29.8878, 19.4662) centre (29.8958, 19.4903) ccw
  arc A1376 (25.9922, 19.8556) -> (25.9762, 19.9038) centre (25.9842, 19.8797) ccw
  arc A1377 (28.4988, 20.3087) -> (28.5496, 20.3087) centre (28.5242, 20.3087) ccw
  arc A1378 (28.5162, 19.0767) -> (28.5322, 19.1249) centre (28.5242, 19.1008) ccw
  arc A1379 (40.0558, 20.3454) -> (40.0558, 20.2946) centre (40.0558, 20.32) ccw
  arc A1380 (28.5322, 19.8556) -> (28.5162, 19.9038) centre (28.5242, 19.8797) ccw
  arc A1381 (27.8567, 20.8429) -> (27.8935, 20.878) centre (27.8751, 20.8605) ccw
  arc A1382 (41.1988, 21.8637) -> (41.2496, 21.8637) centre (41.2242, 21.8637) ccw
  line L425 (25.6921, 19.7824) -> (25.6921, 19.1982)
  arc A1383 (41.2242, 20.9437) -> (41.2242, 20.9945) centre (41.2242, 20.9691) ccw
  arc A1384 (25.9762, 19.0767) -> (25.9922, 19.1249) centre (25.9842, 19.1008) ccw
  arc A1385 (24.8238, 19.5144) -> (24.8078, 19.4662) centre (24.8158, 19.4903) ccw
  arc A1386 (40.8996, 22.2137) -> (40.8996, 22.1629) centre (40.8996, 22.1883) ccw
  arc A1387 (23.0547, 21.0086) -> (23.0547, 21.0594) centre (23.0547, 21.034) ccw
  arc A1388 (27.6479, 20.9832) -> (27.6479, 20.9324) centre (27.6479, 20.9578) ccw
  arc A1389 (28.2067, 19.1982) -> (28.2575, 19.1982) centre (28.2321, 19.1982) ccw
  arc A1390 (41.2496, 21.8637) -> (41.1988, 21.8637) centre (41.2242, 21.8637) ccw
  arc A1391 (25.7175, 19.7824) -> (25.6667, 19.7824) centre (25.6921, 19.7824) ccw
  line L426 (27.8751, 20.8605) -> (28.5242, 20.3087)
  arc A1392 (28.5077, 20.2894) -> (28.5407, 20.3281) centre (28.5242, 20.3087) ccw
  arc A1393 (28.2575, 19.7824) -> (28.2067, 19.7824) centre (28.2321, 19.7824) ccw
  arc A1394 (31.0562, 19.0767) -> (31.0722, 19.1249) centre (31.0642, 19.1008) ccw
  arc A1395 (25.0556, 20.2928) -> (25.0953, 20.3246) centre (25.0755, 20.3087) ccw
  arc A1396 (23.3793, 19.4649) -> (23.3793, 19.5157) centre (23.3793, 19.4903) ccw
  line L427 (24.8158, 20.6333) -> (25.9842, 20.6333)
  line L428 (25.9842, 20.3087) -> (25.9842, 20.9578)
  arc A1397 (40.3804, 22.1629) -> (40.3804, 22.2137) centre (40.3804, 22.1883) ccw
  arc A1398 (24.8158, 20.6587) -> (24.8158, 20.6079) centre (24.8158, 20.6333) ccw
  line L429 (28.5242, 19.1008) -> (27.3558, 19.4903)
  arc A1399 (23.0152, 19.8797) -> (22.9644, 19.8797) centre (22.9898, 19.8797) ccw
  line L430 (41.2242, 21.5392) -> (40.0558, 21.5392)
  arc A1400 (27.3638, 19.5144) -> (27.3478, 19.4662) centre (27.3558, 19.4903) ccw
  arc A1401 (40.0812, 21.8637) -> (40.0304, 21.8637) centre (40.0558, 21.8637) ccw
  line L431 (40.3804, 22.1883) -> (40.8996, 22.1883)
  arc A1402 (25.6667, 19.1982) -> (25.7175, 19.1982) centre (25.6921, 19.1982) ccw
  arc A1403 (24.8356, 20.6491) -> (24.796, 20.6174) centre (24.8158, 20.6333) ccw
  line L432 (27.3558, 19.4903) -> (28.5242, 19.8797)
  arc A1404 (41.2365, 20.9469) -> (41.2119, 20.9913) centre (41.2242, 20.9691) ccw
  arc A1405 (26.0096, 20.9578) -> (25.9588, 20.9578) centre (25.9842, 20.9578) ccw
  line L433 (28.2321, 19.7824) -> (28.2321, 19.1982)
  arc A1406 (27.8751, 20.8605) -> (27.6479, 20.9578) centre (27.648, 20.6441) ccw
  line L434 (24.8158, 19.4903) -> (25.9842, 19.8797)
  arc A1407 (27.6479, 20.9578) -> (27.3558, 20.6657) centre (27.6479, 20.6657) ccw
  line L435 (32.7604, 20.931) -> (33.0849, 20.931)
  arc A1408 (32.7604, 20.9564) -> (32.7604, 20.9056) centre (32.7604, 20.931) ccw
  arc A1409 (31.0896, 20.6333) -> (31.0388, 20.6333) centre (31.0642, 20.6333) ccw
  arc A1410 (32.7604, 20.2565) -> (32.7604, 20.3073) centre (32.7604, 20.2819) ccw
  arc A1411 (33.6042, 20.4117) -> (33.0849, 20.931) centre (33.0849, 20.4117) ccw
  arc A1412 (30.3897, 20.4385) -> (30.4405, 20.4385) centre (30.4151, 20.4385) ccw
  arc A1413 (32.4612, 19.4254) -> (32.4104, 19.4254) centre (32.4358, 19.4254) ccw
  arc A1414 (40.3804, 22.1883) -> (40.0558, 21.8637) centre (40.3804, 21.8637) ccw
  arc A1415 (27.6076, 20.2845) -> (27.6233, 20.3329) centre (27.6155, 20.3087) ccw
  arc A1416 (35.3004, 19.7499) -> (34.9758, 19.4254) centre (35.3004, 19.4253) ccw
  arc A1417 (34.9504, 19.1008) -> (35.0012, 19.1008) centre (34.9758, 19.1008) ccw
  arc A1418 (30.7467, 19.1982) -> (30.7975, 19.1982) centre (30.7721, 19.1982) ccw
  arc A1419 (40.8996, 22.1629) -> (40.8996, 22.2137) centre (40.8996, 22.1883) ccw
  arc A1420 (27.3478, 19.5144) -> (27.3638, 19.4662) centre (27.3558, 19.4903) ccw
  arc A1421 (32.4358, 19.1262) -> (32.4358, 19.0754) centre (32.4358, 19.1008) ccw
  arc A1422 (32.4104, 19.4254) -> (32.4612, 19.4254) centre (32.4358, 19.4254) ccw
  arc A1423 (32.8253, 20.2819) -> (33.0849, 20.5415) centre (32.8253, 20.5415) ccw
  line L436 (33.6042, 19.1008) -> (32.4358, 19.1008)
  arc A1424 (29.8878, 19.5144) -> (29.9038, 19.4662) centre (29.8958, 19.4903) ccw
  arc A1425 (32.8253, 20.3073) -> (32.8253, 20.2565) centre (32.8253, 20.2819) ccw
  arc A1426 (33.1103, 20.5415) -> (33.0595, 20.5415) centre (33.0849, 20.5415) ccw
  arc A1427 (32.8253, 20.2565) -> (32.8253, 20.3073) centre (32.8253, 20.2819) ccw
  line L437 (40.0558, 21.5392) -> (40.0558, 21.8637)
  arc A1428 (31.0642, 20.6333) -> (30.4151, 20.6333) centre (30.7396, 20.6333) ccw
  line L438 (31.0642, 20.3087) -> (31.0642, 20.6333)
  line L439 (33.6042, 19.4254) -> (33.6042, 19.1008)
  arc A1429 (27.3558, 20.6657) -> (27.6154, 20.3087) centre (27.731, 20.6657) ccw
  line L440 (41.2242, 21.8637) -> (41.2242, 21.5392)
  line L441 (29.8958, 19.4903) -> (31.0642, 19.8797)
  line L442 (30.4151, 20.6982) -> (30.4151, 20.4385)
  arc A1430 (31.0388, 20.6333) -> (31.0896, 20.6333) centre (31.0642, 20.6333) ccw
  arc A1431 (30.4405, 20.6982) -> (30.3897, 20.6982) centre (30.4151, 20.6982) ccw
  arc A1432 (33.6042, 19.4254) -> (33.2796, 19.7499) centre (33.2796, 19.4253) ccw
  arc A1433 (33.0595, 20.5415) -> (33.1103, 20.5415) centre (33.0849, 20.5415) ccw
  arc A1434 (32.7604, 19.7499) -> (32.4358, 19.4254) centre (32.7604, 19.4253) ccw
  arc A1435 (40.0304, 21.5392) -> (40.0812, 21.5392) centre (40.0558, 21.5392) ccw
  arc A1436 (30.4151, 20.6982) -> (29.8958, 20.6982) centre (30.1554, 20.6982) ccw
  arc A1437 (32.7604, 20.3073) -> (32.7604, 20.2565) centre (32.7604, 20.2819) ccw
  line L443 (32.7604, 19.7499) -> (33.2796, 19.7499)
  arc A1438 (33.5788, 19.1008) -> (33.6296, 19.1008) centre (33.6042, 19.1008) ccw
  line L444 (34.9758, 19.1008) -> (34.9758, 19.4254)
  arc A1439 (31.0722, 19.8556) -> (31.0562, 19.9038) centre (31.0642, 19.8797) ccw
  arc A1440 (30.3897, 20.6982) -> (30.4405, 20.6982) centre (30.4151, 20.6982) ccw
  arc A1441 (28.5496, 20.9578) -> (28.4988, 20.9578) centre (28.5242, 20.9578) ccw
  arc A1442 (33.2796, 19.7753) -> (33.2796, 19.7245) centre (33.2796, 19.7499) ccw
  arc A1443 (29.8704, 20.6982) -> (29.9212, 20.6982) centre (29.8958, 20.6982) ccw
  arc A1444 (32.4104, 19.1008) -> (32.4612, 19.1008) centre (32.4358, 19.1008) ccw
  arc A1445 (32.7604, 19.7245) -> (32.7604, 19.7753) centre (32.7604, 19.7499) ccw
  arc A1446 (33.0849, 20.9056) -> (33.0849, 20.9564) centre (33.0849, 20.931) ccw
  arc A1447 (29.8704, 20.3087) -> (29.9212, 20.3087) centre (29.8958, 20.3087) ccw
  arc A1448 (32.7604, 19.7753) -> (32.7604, 19.7245) centre (32.7604, 19.7499) ccw
  arc A1449 (30.7975, 19.7824) -> (30.7467, 19.7824) centre (30.7721, 19.7824) ccw
  line L445 (29.8958, 20.3087) -> (29.8958, 20.6982)
  line L446 (30.7721, 19.7824) -> (30.7721, 19.1982)
  arc A1450 (33.2796, 19.7245) -> (33.2796, 19.7753) centre (33.2796, 19.7499) ccw
  arc A1451 (31.0388, 20.3087) -> (31.0896, 20.3087) centre (31.0642, 20.3087) ccw
  arc A1452 (30.3897, 20.6333) -> (30.4405, 20.6333) centre (30.4151, 20.6333) ccw
  arc A1453 (32.7604, 20.931) -> (32.7604, 20.2819) centre (32.7604, 20.6065) ccw
  arc A1454 (35.0012, 19.4254) -> (34.9504, 19.4254) centre (34.9758, 19.4254) ccw
  line L447 (33.0849, 20.931) -> (33.0849, 20.5415)
  arc A1455 (29.9212, 20.6982) -> (29.8704, 20.6982) centre (29.8958, 20.6982) ccw
  line L448 (32.4358, 19.1008) -> (32.4358, 19.4254)
  arc A1456 (32.7604, 20.9056) -> (32.7604, 20.9564) centre (32.7604, 20.931) ccw
  arc A1457 (33.6296, 19.4254) -> (33.5788, 19.4254) centre (33.6042, 19.4254) ccw
  line L449 (36.1442, 20.2819) -> (36.1442, 20.931)
  arc A1458 (35.1269, 21.9995) -> (35.1492, 21.9538) centre (35.138, 21.9767) ccw
  arc A1459 (34.9956, 20.6223) -> (34.956, 20.5906) centre (34.9758, 20.6065) ccw
  arc A1460 (35.2513, 22.0289) -> (35.2196, 21.9893) centre (35.2355, 22.0091) ccw
  arc A1461 (35.1492, 21.5451) -> (35.1269, 21.4994) centre (35.138, 21.5223) ccw
  arc A1462 (35.9737, 21.5463) -> (35.9902, 21.4982) centre (35.9819, 21.5222) ccw
  arc A1463 (35.9902, 22.0007) -> (35.9737, 21.9526) centre (35.9819, 21.9767) ccw
  arc A1464 (38.2552, 25.0613) -> (38.2044, 25.0613) centre (38.2298, 25.0613) ccw
  line L450 (36.1442, 19.4254) -> (36.1442, 19.1008)
  arc A1465 (33.1103, 20.931) -> (33.0595, 20.931) centre (33.0849, 20.931) ccw
  arc A1466 (36.1188, 19.1008) -> (36.1696, 19.1008) centre (36.1442, 19.1008) ccw
  arc A1467 (35.8196, 19.7753) -> (35.8196, 19.7245) centre (35.8196, 19.7499) ccw
  arc A1468 (38.2552, 23.7659) -> (38.2044, 23.7659) centre (38.2298, 23.7659) ccw
  line L451 (38.2298, 24.2824) -> (38.2298, 25.0613)
  arc A1469 (33.5788, 19.4254) -> (33.6296, 19.4254) centre (33.6042, 19.4254) ccw
  arc A1470 (34.9758, 19.1262) -> (34.9758, 19.0754) centre (34.9758, 19.1008) ccw
  arc A1471 (36.1442, 19.0754) -> (36.1442, 19.1262) centre (36.1442, 19.1008) ccw
  line L452 (38.2298, 20.3962) -> (38.2298, 21.1751)
  line L453 (35.3004, 19.7499) -> (35.8196, 19.7499)
  arc A1472 (35.56, 21.4503) -> (35.56, 21.3995) centre (35.56, 21.4249) ccw
  arc A1473 (36.1188, 20.2819) -> (36.1696, 20.2819) centre (36.1442, 20.2819) ccw
  arc A1474 (35.8687, 21.47) -> (35.9004, 21.5096) centre (35.8845, 21.4898) ccw
  arc A1475 (38.2552, 19.8797) -> (38.2044, 19.8797) centre (38.2298, 19.8797) ccw
  arc A1476 (38.2044, 24.2824) -> (38.2552, 24.2824) centre (38.2298, 24.2824) ccw
  line L454 (38.2298, 22.987) -> (38.2298, 23.7659)
  arc A1477 (33.0849, 20.9564) -> (33.0849, 20.9056) centre (33.0849, 20.931) ccw
  arc A1478 (35.56, 22.074) -> (35.1381, 21.9766) centre (35.5601, 21.1113) ccw
  arc A1479 (35.0012, 21.7494) -> (34.9504, 21.7494) centre (34.9758, 21.7494) ccw
  arc A1480 (33.6042, 19.0754) -> (33.6042, 19.1262) centre (33.6042, 19.1008) ccw
  arc A1481 (34.9758, 20.6319) -> (34.9758, 20.5811) centre (34.9758, 20.6065) ccw
  arc A1482 (33.5788, 20.4117) -> (33.6296, 20.4117) centre (33.6042, 20.4117) ccw
  line L455 (34.9758, 20.6065) -> (36.1442, 20.6065)
  arc A1483 (34.9504, 21.7494) -> (35.0012, 21.7494) centre (34.9758, 21.7494) ccw
  arc A1484 (38.2044, 20.3962) -> (38.2552, 20.3962) centre (38.2298, 20.3962) ccw
  arc A1485 (36.1442, 21.7494) -> (35.9819, 21.9766) centre (35.904, 21.7494) ccw
  arc A1486 (35.1381, 21.9766) -> (34.9758, 21.7494) centre (35.216, 21.7494) ccw
  arc A1487 (36.1696, 21.7494) -> (36.1188, 21.7494) centre (36.1442, 21.7494) ccw
  arc A1488 (36.1442, 20.5811) -> (36.1442, 20.6319) centre (36.1442, 20.6065) ccw
  arc A1489 (35.1463, 21.9526) -> (35.1298, 22.0007) centre (35.138, 21.9766) ccw
  arc A1490 (35.9931, 21.4994) -> (35.9708, 21.5451) centre (35.982, 21.5223) ccw
  line L456 (32.8253, 20.2819) -> (32.7604, 20.2819)
  arc A1491 (35.56, 21.4249) -> (35.9819, 21.5223) centre (35.5599, 22.3876) ccw
  arc A1492 (36.1442, 19.4254) -> (35.8196, 19.7499) centre (35.8196, 19.4253) ccw
  arc A1493 (35.3004, 19.7753) -> (35.3004, 19.7245) centre (35.3004, 19.7499) ccw
  arc A1494 (35.56, 22.0994) -> (35.56, 22.0486) centre (35.56, 22.074) ccw
  line L457 (38.2298, 19.1008) -> (38.2298, 19.8797)
  arc A1495 (34.9504, 19.4254) -> (35.0012, 19.4254) centre (34.9758, 19.4254) ccw
  arc A1496 (36.1696, 20.931) -> (36.1188, 20.931) centre (36.1442, 20.931) ccw
  line L458 (76.7842, 35.6108) -> (75.6158, 36.0003)
  arc A1497 (35.9819, 21.5223) -> (36.1442, 21.7494) centre (35.9041, 21.7494) ccw
  arc A1498 (35.8196, 19.7245) -> (35.8196, 19.7753) centre (35.8196, 19.7499) ccw
  arc A1499 (36.1188, 21.7494) -> (36.1696, 21.7494) centre (36.1442, 21.7494) ccw
  arc A1500 (35.56, 22.0486) -> (35.56, 22.0994) centre (35.56, 22.074) ccw
  arc A1501 (75.6238, 36.0244) -> (75.6078, 35.9762) centre (75.6158, 36.0003) ccw
  arc A1502 (35.1381, 21.5223) -> (35.56, 21.4249) centre (35.5601, 22.3876) ccw
  arc A1503 (34.9758, 21.7494) -> (35.1381, 21.5223) centre (35.2159, 21.7494) ccw
  arc A1504 (35.1298, 21.4982) -> (35.1463, 21.5463) centre (35.1381, 21.5222) ccw
  line L459 (38.2298, 21.6916) -> (38.2298, 22.4705)
  arc A1505 (35.9819, 21.9766) -> (35.56, 22.074) centre (35.5599, 21.1113) ccw
  arc A1506 (36.1696, 19.4254) -> (36.1188, 19.4254) centre (36.1442, 19.4254) ccw
  arc A1507 (38.2044, 19.1008) -> (38.2552, 19.1008) centre (38.2298, 19.1008) ccw
  arc A1508 (35.9708, 21.9538) -> (35.9931, 21.9995) centre (35.9819, 21.9767) ccw
  arc A1509 (36.1188, 19.4254) -> (36.1696, 19.4254) centre (36.1442, 19.4254) ccw
  line L460 (36.1442, 19.1008) -> (34.9758, 19.1008)
  arc A1510 (75.9404, 40.6301) -> (75.6158, 40.3056) centre (75.9404, 40.3055) ccw
  arc A1511 (75.5904, 40.3056) -> (75.6412, 40.3056) centre (75.6158, 40.3056) ccw
  arc A1512 (75.6228, 37.1028) -> (75.6088, 37.0539) centre (75.6158, 37.0784) ccw
  arc A1513 (75.6412, 40.3056) -> (75.5904, 40.3056) centre (75.6158, 40.3056) ccw
  arc A1514 (75.7335, 39.407) -> (75.6928, 39.4374) centre (75.7132, 39.4222) ccw
  arc A1515 (76.4596, 40.6555) -> (76.4596, 40.6047) centre (76.4596, 40.6301) ccw
  arc A1516 (76.4992, 36.8187) -> (76.55, 36.8187) centre (76.5246, 36.8187) ccw
  arc A1517 (76.2649, 37.2985) -> (76.2649, 37.2477) centre (76.2649, 37.2731) ccw
  line L461 (75.6158, 36.0003) -> (76.7842, 36.3897)
  arc A1518 (75.9404, 40.6047) -> (75.9404, 40.6555) centre (75.9404, 40.6301) ccw
  line L462 (76.914, 37.9123) -> (75.486, 38.4316)
  arc A1519 (76.0803, 39.0124) -> (76.1249, 38.9881) centre (76.1026, 39.0003) ccw
  arc A1520 (38.2552, 21.1751) -> (38.2044, 21.1751) centre (38.2298, 21.1751) ccw
  line L463 (76.2649, 37.2731) -> (76.7842, 37.2731)
  arc A1521 (76.55, 37.4678) -> (76.4992, 37.4678) centre (76.5246, 37.4678) ccw
  arc A1522 (75.6078, 36.0244) -> (75.6238, 35.9762) centre (75.6158, 36.0003) ccw
  arc A1523 (75.8754, 38.8705) -> (76.1026, 39.0003) centre (75.8754, 39.1342) ccw
  arc A1524 (76.7588, 39.2275) -> (76.8096, 39.2275) centre (76.7842, 39.2275) ccw
  arc A1525 (76.8096, 39.2275) -> (76.7588, 39.2275) centre (76.7842, 39.2275) ccw
  arc A1526 (35.3004, 19.7245) -> (35.3004, 19.7753) centre (35.3004, 19.7499) ccw
  line L464 (76.2974, 39.3573) -> (76.1026, 39.0003)
  arc A1527 (38.2044, 21.6916) -> (38.2552, 21.6916) centre (38.2298, 21.6916) ccw
  arc A1528 (76.6219, 38.838) -> (76.7842, 39.2275) centre (76.2357, 39.2275) ccw
  arc A1529 (35.2156, 20.266) -> (35.2553, 20.2978) centre (35.2355, 20.2819) ccw
  arc A1530 (75.8754, 38.8959) -> (75.8754, 38.8451) centre (75.8754, 38.8705) ccw
  line L465 (76.7842, 39.981) -> (75.6158, 39.981)
  line L466 (75.6158, 41.4867) -> (76.7842, 41.8761)
  line L467 (75.6158, 37.0784) -> (76.5246, 36.8187)
  arc A1531 (76.7922, 41.852) -> (76.7762, 41.9002) centre (76.7842, 41.8761) ccw
  arc A1532 (75.4947, 38.4555) -> (75.4773, 38.4077) centre (75.486, 38.4316) ccw
  arc A1533 (75.6158, 39.1301) -> (75.8754, 38.8705) centre (75.8754, 39.1301) ccw
  arc A1534 (76.9053, 37.8884) -> (76.9227, 37.9362) centre (76.914, 37.9123) ccw
  arc A1535 (75.6412, 39.1301) -> (75.5904, 39.1301) centre (75.6158, 39.1301) ccw
  line L468 (35.8846, 21.4898) -> (35.2354, 22.0091)